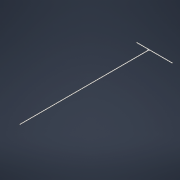
# Autodesk Inventor part: FloorStripe
Saved by Autodesk Inventor 2021 (Build 250183000, 183)
## iProperties
Created: 2021-01-31
Part Number: FloorStripe
Material: Generic
Document SubType Name: Modeling
Designer: argon
Density: 1 g/cm^3
Appearance: Default
Author: argon
Autodesk Inventor part; units mm, degrees
ref_plane "YZ Plane" through (0, 0, 0) normal (1, 0, 0) x (0, 1, 0)
ref_plane "XZ Plane" through (0, 0, 0) normal (0, 1, 0) x (-1, 0, 0)
ref_plane "XY Plane" through (0, 0, 0) normal (0, 0, 1) x (1, 0, 0)
sketch "Sketch1" plane through (0, 0, 0) normal (0, 1, 0) x (-1, 0, 0)
  line L0 (1974.0363, 0) -> (1974.0363, -11147.7438)
  line L1 (1974.0363, -11147.7438) -> (2074.0363, -11147.7438)
  line L2 (2074.0363, -11147.7438) -> (2074.0363, 0)
  line L3 (0, 0) -> (0, -12000)
  line L4 (3138.0727, -11247.7438) -> (0, -11247.7438)
  line L5 (0, -11247.7438) -> (0, -11147.7438)
  line L6 (0, -11147.7438) -> (3138.0727, -11147.7438)
  line L7 (3138.0727, -11147.7438) -> (3138.0727, -11247.7438)
  line L8 (3138.0727, 0) -> (3138.0727, -12000)
  line L9 (2074.0363, 0) -> (1974.0363, 0)
  point P0 (1974.0363, -9581.3845)
  point P1 (2074.0363, -9581.3845)
  dimension "d0" = 100
  constraints: 20 end point, 4 point on line, 3 parallel, 2 horizontal, 2 perpendicular, 1 collinear
  measures "d0" distance between parallel lines of L0 L2
extrude "Extrusion1" add sketch "Sketch1" along normal blind 5
fillet "Fillet1" radius 100 2 edges at (-1974.0363, 2.5, -11147.7438) (-2074.0363, 2.5, -11147.7438)
body "Solid1"
